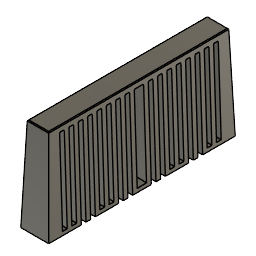
RISERbars-2 (Autodesk Fusion 360 design; units mm, degrees)
part number: 2026-05-24-12-34-57-547
Autodesk Fusion 360 part; units mm, degrees
sketch "Sketch1" plane through (0, 0, 0) normal (0, 0, 1) x (1, 0, 0)
  line L0 (0, 0) -> (30, 0)
  line L1 (30, 0) -> (30, 200)
  line L2 (30, 200) -> (0, 200)
  line L3 (0, 200) -> (0, 0)
  dimension "d1" = 200
  dimension "d2" = 30
  constraint horizontal L0
  constraint vertical L1
  constraint horizontal L2
  constraint vertical L3
  constraint coincident L0.start L3.end
  measures "d1" distance of L0.start L2.end
  measures "d2" distance of L1 L3
extrude "Extrude1" add sketch "Sketch1" along normal blind 100 draft -2
sketch "Sketch3" plane through (0, 0, 0) normal (-0.999391, 0, 0.034899) x (0, -1, 0)
  line L0 (-200, 0) -> (0, 0)
  line L1 (0, 0) -> (-3.4921, 100.061)
  line L2 (-3.4921, 100.061) -> (-196.5079, 100.061)
  line L3 (-196.5079, 100.061) -> (-200, 0)
  line L4 (-190, -45) -> (-195, -45)
  line L5 (-185, 95.061) -> (-180, 95.061)
  line L6 (-180, 95.061) -> (-180, 5)
  line L7 (-180, 5) -> (-185, 5)
  line L8 (-185, 5) -> (-185, 95.061)
  line L9 (-100, -24.2612) -> (-100, 190) construction
  line L10 (-177.5, 100.061) -> (-177.5, -9.0071)
  line L11 (-160, -45) -> (-160, 95)
  line L12 (-165, -45) -> (-160, -45)
  line L13 (-165, 95) -> (-165, -45)
  line L14 (-160, 95) -> (-165, 95)
  line L15 (-170, 95.061) -> (-175, 95.061)
  line L16 (-170, 5) -> (-170, 95.061)
  line L17 (-175, 95.061) -> (-175, 5)
  line L18 (-175, 5) -> (-170, 5)
  line L19 (-157.5, 158.7184) -> (-157.5, -20.0117)
  line L20 (-140, 95.061) -> (-140, 5)
  line L21 (-145, 5) -> (-145, 95.061)
  line L22 (-145, 95.061) -> (-140, 95.061)
  line L23 (-140, 5) -> (-145, 5)
  line L24 (-155, 95) -> (-150, 95)
  line L25 (-150, 95) -> (-150, -45)
  line L26 (-155, -45) -> (-155, 95)
  line L27 (-150, -45) -> (-155, -45)
  line L28 (-50, -45) -> (-45, -45)
  line L29 (-25, 5) -> (-30, 5)
  line L30 (-60, 5) -> (-55, 5)
  line L31 (-55, 5) -> (-55, 95.061)
  line L32 (-10, -45) -> (-5, -45)
  line L33 (-45, -45) -> (-45, 95)
  line L34 (-25, 95.061) -> (-25, 5)
  line L35 (-50, 95) -> (-50, -45)
  line L36 (-40, -45) -> (-40, 95)
  line L37 (-40, 95) -> (-35, 95)
  line L38 (-45, 95) -> (-50, 95)
  line L39 (-60, 95.061) -> (-60, 5)
  line L40 (-35, -45) -> (-40, -45)
  line L41 (-35, 95) -> (-35, -45)
  line L42 (-20, 5) -> (-15, 5)
  line L43 (-30, 95.061) -> (-25, 95.061)
  line L44 (-15, 95.061) -> (-20, 95.061)
  line L45 (-30, 5) -> (-30, 95.061)
  line L46 (-55, 95.061) -> (-60, 95.061)
  line L47 (-15, 5) -> (-15, 95.061)
  line L48 (-20, 95.061) -> (-20, 5)
  line L49 (-140, 5) -> (-145, 5)
  line L50 (-125, -45) -> (-120, -45)
  line L51 (-130, 95.061) -> (-135, 95.061)
  line L52 (-120, 95) -> (-125, 95)
  line L53 (-125, 95) -> (-125, -45)
  line L54 (-120, -45) -> (-120, 95)
  line L55 (-145, 95.061) -> (-140, 95.061)
  line L56 (-150, -45) -> (-155, -45)
  line L57 (-130, 5) -> (-130, 95.061)
  line L58 (-155, -45) -> (-155, 95)
  line L59 (-140, 95.061) -> (-140, 5)
  line L60 (-145, 5) -> (-145, 95.061)
  line L61 (-155, 95) -> (-150, 95)
  line L62 (-135, 5) -> (-130, 5)
  line L63 (-150, 95) -> (-150, -45)
  line L64 (-135, 95.061) -> (-135, 5)
  line L65 (-117.5, 160.0115) -> (-117.5, -13.2557)
  line L66 (-105, 5) -> (-105, 95.061)
  line L67 (-110, -45) -> (-115, -45)
  line L68 (-110, 95) -> (-110, -45)
  line L69 (-115, -45) -> (-115, 95)
  line L70 (-100, 95.061) -> (-100, 5)
  line L71 (-100, 5) -> (-105, 5)
  line L72 (-105, 95.061) -> (-100, 95.061)
  line L73 (-115, 95) -> (-110, 95)
  line L74 (-80, -45) -> (-80, 95)
  line L75 (-60, 5) -> (-55, 5)
  line L76 (-60, 5) -> (-55, 5)
  line L77 (-35, -45) -> (-40, -45)
  line L78 (-20, 5) -> (-15, 5)
  line L79 (-75, -45) -> (-80, -45)
  line L80 (-55, 5) -> (-55, 95.061)
  line L81 (-55, 5) -> (-55, 95.061)
  line L82 (-55, 95.061) -> (-60, 95.061)
  line L83 (-35, 95) -> (-35, -45)
  line L84 (-45, 95) -> (-50, 95)
  line L85 (-70, 5) -> (-70, 95.061)
  line L86 (-60, 95.061) -> (-60, 5)
  line L87 (-70, 95.061) -> (-65, 95.061)
  line L88 (-50, 95) -> (-50, -45)
  line L89 (-45, -45) -> (-45, 95)
  line L90 (-40, 95) -> (-35, 95)
  line L91 (-75, 95) -> (-75, -45)
  line L92 (-65, 95.061) -> (-65, 5)
  line L93 (-90, -45) -> (-85, -45)
  line L94 (-85, 95) -> (-90, 95)
  line L95 (-20, 95.061) -> (-20, 5)
  line L96 (-30, 5) -> (-30, 95.061)
  line L97 (-30, 95.061) -> (-25, 95.061)
  line L98 (-60, 95.061) -> (-60, 5)
  line L99 (-85, -45) -> (-85, 95)
  line L100 (-25, 5) -> (-30, 5)
  line L101 (-45, -45) -> (-45, 95)
  line L102 (-10, -45) -> (-5, -45)
  line L103 (-50, -45) -> (-45, -45)
  line L104 (-25, 95.061) -> (-25, 5)
  line L105 (-95, 5) -> (-95, 95.061)
  line L106 (-90, 95) -> (-90, -45)
  line L107 (-65, 5) -> (-70, 5)
  line L108 (-15, 5) -> (-15, 95.061)
  line L109 (-50, -45) -> (-45, -45)
  line L110 (-45, 95) -> (-50, 95)
  line L111 (-80, 95) -> (-75, 95)
  line L112 (-55, 95.061) -> (-60, 95.061)
  line L113 (-40, -45) -> (-40, 95)
  line L114 (-15, 95.061) -> (-20, 95.061)
  line L115 (-50, 95) -> (-50, -45)
  line L116 (-95, 95.061) -> (-100, 95.061)
  line L117 (-100, 5) -> (-95, 5)
  dimension "d24" = 5
  dimension "d25" = 5
  dimension "d26" = 5
  dimension "d28" = 2.5
  dimension "d29" = 2.5
  dimension "d30" = 2.5
  constraint horizontal L4
  constraint horizontal L5
  constraint vertical L6
  constraint horizontal L7
  constraint vertical L8
  constraint perpendicular L2 L9
  constraint coincident L2 L10.start
  constraint parallel L6 L10
  constraint symmetric L4.start L10 L12.start
  constraint symmetric L4.end L10 L11.start
  constraint symmetric L5.start L10 L15.start
  constraint symmetric L5.end L10 L15.end
  constraint symmetric L6.end L10 L17.end
  constraint symmetric L7.end L10 L16.start
  constraint parallel L11 L19
  constraint symmetric L11.start L19 L26.start
  constraint symmetric L11.end L19 L24.start
  constraint symmetric L12.start L19 L25.end
  constraint symmetric L13.start L19 L24.end
  constraint symmetric L15.start L19 L21.end
  constraint symmetric L15.end L19 L20.start
  constraint symmetric L16.start L19 L21.start
  constraint symmetric L17.end L19 L20.end
  constraint symmetric L4.start L9 L32.start
  constraint symmetric L4.end L9 L32.end
  constraint symmetric L5.start L9 L44.start
  constraint symmetric L5.end L9 L44.end
  constraint symmetric L6.end L9 L42.start
  constraint symmetric L7.end L9 L42.end
  constraint symmetric L9 L11.start L36.start
  constraint symmetric L9 L11.end L36.end
  constraint symmetric L9 L12.start L40.start
  constraint symmetric L9 L13.start L37.end
  constraint symmetric L9 L15.start L43.start
  constraint symmetric L9 L15.end L34.start
  constraint symmetric L9 L16.start L29.end
  constraint symmetric L9 L17.end L29.start
  constraint symmetric L9 L20.start L39.start
  constraint symmetric L9 L20.end L30.start
  constraint symmetric L9 L21.start L30.end
  constraint symmetric L9 L21.end L31.end
  constraint symmetric L9 L24.start L33.end
  constraint symmetric L9 L24.end L35.start
  constraint symmetric L9 L25.end L28.start
  constraint symmetric L9 L26.start L28.end
  constraint symmetric L4.start L19 L50.start
  constraint symmetric L4.end L19 L50.end
  constraint symmetric L5.start L19 L51.start
  constraint symmetric L5.end L19 L51.end
  constraint symmetric L6.end L19 L62.start
  constraint symmetric L7.end L19 L57.start
  constraint parallel L54 L65
  constraint symmetric L50.start L65 L67.start
  constraint symmetric L52.end L65 L68.start
  constraint symmetric L50.end L65 L67.end
  constraint symmetric L62.start L65 L70.end
  constraint symmetric L57.start L65 L66.start
  constraint symmetric L52.start L65 L69.end
  constraint symmetric L51.end L65 L70.start
  constraint symmetric L51.start L65 L66.end
  constraint symmetric L9 L50.start L79.start
  constraint symmetric L9 L52.end L91.start
  constraint symmetric L9 L50.end L74.start
  constraint symmetric L9 L62.start L92.end
  constraint symmetric L9 L57.start L85.start
  constraint symmetric L9 L52.start L74.end
  constraint symmetric L9 L51.end L87.end
  constraint symmetric L9 L51.start L85.end
  constraint symmetric L9 L70.end L71.start
  constraint symmetric L9 L66.end L105.end
  constraint symmetric L9 L70.start L72.end
  constraint symmetric L9 L66.start L105.start
  constraint symmetric L9 L68.start L94.end
  constraint symmetric L9 L67.start L93.start
  constraint symmetric L9 L67.end L93.end
  constraint symmetric L9 L69.end L94.start
  measures "d24" distance of L2 L5
  measures "d25" distance of L0 L7
  measures "d26" distance of L6 L8
  measures "d28" distance of L6 L10
  measures "d29" distance of L11 L19
  measures "d30" distance of L54 L65
extrude "Extrude5" cut sketch "Sketch3" against normal blind 100 contours L0 L11 L13 L14 | L0 L11 L12 L13 | L0 L24 L25 L26 L58 L61 L63 | L0 L25 L26 L27 L56 L58 L63 | L0 L50 L53 L54 | L0 L52 L53 L54 | L0 L68 L69 L73 | L0 L67 L68 L69 | L0 L36 L40 L41 L77 L83 L113 | L0 L36 L37 L41 L83 L90 L113 | L0 L94 L99 L106 | L0 L93 L99 L106 | L0 L28 L33 L35 L88 L89 L101 L103 L109 L115 | L0 L33 L35 L38 L84 L88 L89 L101 L110 L115 | L0 L74 L91 L111 | L0 L74 L79 L91 | L5 L6 L7 L8 | L15 L16 L17 L18 | L20 L21 L22 L23 L49 L55 L59 L60 | L29 L34 L43 L45 L96 L97 L100 L104 | L30 L31 L39 L46 L75 L76 L80 L81 L82 L86 L98 L112 | L42 L44 L47 L48 L78 L95 L108 L114 | L51 L57 L62 L64 | L66 L70 L71 L72 | L70 L105 L116 L117 | L85 L87 L92 L107
chamfer "Chamfer3" distance 0.8 angle 45 38 edges at (15, 196.5079, 100) (15, 3.4921, 100) (3.4921, 100, 100) (26.5079, 100, 100) (15.0143, 185, 94.5946) (15.0143, 180, 94.5946) (15.0143, 175, 94.5946) (15.0143, 170, 94.5946) (15.0143, 165, 94.5336) (15.0143, 160, 94.5336) (15.0143, 155, 94.5336) (15.0143, 150, 94.5336) (15.0143, 145, 94.5946) (15.0143, 140, 94.5946) (15.0143, 135, 94.5946) (15.0143, 130, 94.5946) (15.0143, 125, 94.5336) (15.0143, 120, 94.5336) (15.0143, 115, 94.5336) (15.0143, 110, 94.5336) (15.0143, 105, 94.5946) (15.0143, 95, 94.5946) (15.0143, 90, 94.5336) (15.0143, 85, 94.5336) (15.0143, 80, 94.5336) (15.0143, 75, 94.5336) (15.0143, 70, 94.5946) (15.0143, 65, 94.5946) (15.0143, 60, 94.5946) (15.0143, 55, 94.5946) (15.0143, 50, 94.5336) (15.0143, 45, 94.5336) (15.0143, 40, 94.5336) (15.0143, 35, 94.5336) (15.0143, 30, 94.5946) (15.0143, 25, 94.5946) (15.0143, 20, 94.5946) (15.0143, 15, 94.5946)
